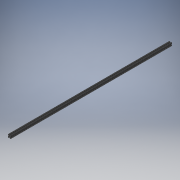
# Autodesk Inventor part: 30-3030-1708-CL
Saved by Autodesk Inventor 2019 (Build 230136000, 136)
## iProperties
Created: 2023-03-27
Part Number: 30-3030-1708-CL
Material: Generic
Catalog Web Link: www.cadenas.de
Description: 30-3030, 30-3030-Black-T-Slotted Profile - 30 Series
Vendor: 8020
Document SubType Name: Modeling
Designer: psAdmin
Manufacturer: 8020
Mass: 538.109 g
Surface Area: 5681.46 cm^2
Volume: 538.109 cm^3
Density: 1 g/cm^3
Appearance: PSOLRGB-191-191-191
Category: PARTsolutions
Company: 8020
Title: 30-3030-1708
Author: Cadenas PARTsolutions
Comments: T-Slotted Profile - 30 Series
PSOL_IDENT_0: {$CADENAS_DATA/23d-libs/8020/metric/profiles/30_series/30_3030.prj},192 {VTYP=3D},{NB=30-3030-1708-C
PSOL_IDENT_1: L},{LINA=30-3030-1708},{NN=30-3030, 30-3030-Black},{DATE=31.07.2020 09:21:33},{GEOMDATE=01.11.2018 1
PSOL_IDENT_2: 7:26:00},{VERSION=},{LINEID=10},{WBVAR=FIN,LS,L},{WBNUMERIC=L}  {NB=30-3030-1708-CL},{LINA=30-3030-1
PSOL_IDENT_3: 708},{KT=DUMMY},{PN=30-3030-1708},{PN1=30-3030},{FIN=CA},{LS=-CL},{L=1708.00},{SERIES=30-3030},{MAT=
PSOL_IDENT_4: 6105-T5 Aluminum},{W=0.9376},{LALG=[25:6000/0.05]},{MIX=2.7222},{MIY=2.7222},{EA=3.0877},{COLOR=.75,
PSOL_IDENT_5: .75,.75}
NB: 30-3030-1708-CL
NN: 30-3030, 30-3030-Black
NT: T-Slotted Profile - 30 Series
NBSYN: $PN.$LS.
LINA: 30-3030-1708
CATALOG: 80/20
PN: 30-3030-1708
FIN: Clear Anodize
LS: Custom Length
L: 1708
SERIES: 30-3030
MAT: 6105-T5 Aluminum
W: 0.9376
MIX: 2.7222
MIY: 2.7222
EA: 3.0877
SUPPLIER: 8020
ARTICLENO: 30-3030-1708-CL
BOMINFO: 30-3030-1708
CREATOR: CADENAS GmbH
Autodesk Inventor part; units mm, degrees
ref_plane "YZ Plane" through (0, 0, 0) normal (1, 0, 0) x (0, 1, 0)
ref_plane "XZ Plane" through (0, 0, 0) normal (0, 1, 0) x (-1, 0, 0)
ref_plane "XY Plane" through (0, 0, 0) normal (0, 0, 1) x (1, 0, 0)
sketch "Sketch_1" plane through (0, 0, 0) normal (0, 0, 1) x (1, 0, 0)
  arc A0 (-15, -13) -> (-13, -15) centre (-13, -13) ccw
  line L0 (-13, -15) -> (-4.508, -15)
  arc A1 (-4.508, -15) -> (-4, -14.492) centre (-4.508, -14.492) ccw
  line L1 (-4, -14.492) -> (-4, -13.251)
  arc A2 (-4, -13.251) -> (-4.508, -12.743) centre (-4.508, -13.251) ccw
  line L2 (-4.508, -12.743) -> (-7.742, -12.743)
  arc A3 (-8.25, -12.235) -> (-7.742, -12.743) centre (-7.742, -12.235) ccw
  line L3 (-8.25, -12.235) -> (-8.25, -10.2642)
  arc A4 (-8.1012, -9.905) -> (-8.25, -10.2642) centre (-7.742, -10.2642) ccw
  line L4 (-8.1012, -9.905) -> (-4.1795, -5.9833)
  arc A5 (-3.8203, -5.8345) -> (-4.1795, -5.9833) centre (-3.8203, -6.3425) ccw
  line L5 (-3.8203, -5.8345) -> (-0.949, -5.8345)
  line L6 (-0.949, -5.8345) -> (0, -5.325)
  line L7 (0, -5.325) -> (0.949, -5.8345)
  line L8 (0.949, -5.8345) -> (3.8216, -5.8345)
  arc A6 (4.1808, -5.9833) -> (3.8216, -5.8345) centre (3.8216, -6.3425) ccw
  line L9 (4.1808, -5.9833) -> (8.1012, -9.9037)
  arc A7 (8.25, -10.2629) -> (8.1012, -9.9037) centre (7.742, -10.2629) ccw
  line L10 (8.25, -10.2629) -> (8.25, -12.235)
  arc A8 (7.742, -12.743) -> (8.25, -12.235) centre (7.742, -12.235) ccw
  line L11 (7.742, -12.743) -> (4.508, -12.743)
  arc A9 (4.508, -12.743) -> (4, -13.251) centre (4.508, -13.251) ccw
  line L12 (4, -13.251) -> (4, -14.492)
  arc A10 (4, -14.492) -> (4.508, -15) centre (4.508, -14.492) ccw
  line L13 (4.508, -15) -> (13, -15)
  arc A11 (13, -15) -> (15, -13) centre (13, -13) ccw
  line L14 (15, -13) -> (15, -4.508)
  arc A12 (15, -4.508) -> (14.492, -4) centre (14.492, -4.508) ccw
  line L15 (14.492, -4) -> (13.251, -4)
  arc A13 (13.251, -4) -> (12.743, -4.508) centre (13.251, -4.508) ccw
  line L16 (12.743, -4.508) -> (12.743, -7.742)
  arc A14 (12.235, -8.25) -> (12.743, -7.742) centre (12.235, -7.742) ccw
  line L17 (12.235, -8.25) -> (10.2642, -8.25)
  arc A15 (9.905, -8.1012) -> (10.2642, -8.25) centre (10.2642, -7.742) ccw
  line L18 (9.905, -8.1012) -> (5.9833, -4.1795)
  arc A16 (5.8345, -3.8203) -> (5.9833, -4.1795) centre (6.3425, -3.8203) ccw
  line L19 (5.8345, -3.8203) -> (5.8345, -0.949)
  line L20 (5.8345, -0.949) -> (5.325, 0)
  line L21 (5.325, 0) -> (5.8345, 0.949)
  line L22 (5.8345, 0.949) -> (5.8345, 3.8216)
  arc A17 (5.9833, 4.1808) -> (5.8345, 3.8216) centre (6.3425, 3.8216) ccw
  line L23 (5.9833, 4.1808) -> (9.9037, 8.1012)
  arc A18 (10.2629, 8.25) -> (9.9037, 8.1012) centre (10.2629, 7.742) ccw
  line L24 (10.2629, 8.25) -> (12.235, 8.25)
  arc A19 (12.743, 7.742) -> (12.235, 8.25) centre (12.235, 7.742) ccw
  line L25 (12.743, 7.742) -> (12.743, 4.508)
  arc A20 (12.743, 4.508) -> (13.251, 4) centre (13.251, 4.508) ccw
  line L26 (13.251, 4) -> (14.492, 4)
  arc A21 (14.492, 4) -> (15, 4.508) centre (14.492, 4.508) ccw
  line L27 (15, 4.508) -> (15, 13)
  arc A22 (15, 13) -> (13, 15) centre (13, 13) ccw
  line L28 (13, 15) -> (4.508, 15)
  arc A23 (4.508, 15) -> (4, 14.492) centre (4.508, 14.492) ccw
  line L29 (4, 14.492) -> (4, 13.251)
  arc A24 (4, 13.251) -> (4.508, 12.743) centre (4.508, 13.251) ccw
  line L30 (4.508, 12.743) -> (7.742, 12.743)
  arc A25 (8.25, 12.235) -> (7.742, 12.743) centre (7.742, 12.235) ccw
  line L31 (8.25, 12.235) -> (8.25, 10.2642)
  arc A26 (8.1012, 9.905) -> (8.25, 10.2642) centre (7.742, 10.2642) ccw
  line L32 (8.1012, 9.905) -> (4.1795, 5.9833)
  arc A27 (3.8203, 5.8345) -> (4.1795, 5.9833) centre (3.8203, 6.3425) ccw
  line L33 (3.8203, 5.8345) -> (0.949, 5.8345)
  line L34 (0.949, 5.8345) -> (0, 5.325)
  line L35 (0, 5.325) -> (-0.949, 5.8345)
  line L36 (-0.949, 5.8345) -> (-3.8216, 5.8345)
  arc A28 (-4.1808, 5.9833) -> (-3.8216, 5.8345) centre (-3.8216, 6.3425) ccw
  line L37 (-4.1808, 5.9833) -> (-8.1012, 9.9037)
  arc A29 (-8.25, 10.2629) -> (-8.1012, 9.9037) centre (-7.742, 10.2629) ccw
  line L38 (-8.25, 10.2629) -> (-8.25, 12.235)
  arc A30 (-7.742, 12.743) -> (-8.25, 12.235) centre (-7.742, 12.235) ccw
  line L39 (-7.742, 12.743) -> (-4.508, 12.743)
  arc A31 (-4.508, 12.743) -> (-4, 13.251) centre (-4.508, 13.251) ccw
  line L40 (-4, 13.251) -> (-4, 14.492)
  arc A32 (-4, 14.492) -> (-4.508, 15) centre (-4.508, 14.492) ccw
  line L41 (-4.508, 15) -> (-13, 15)
  arc A33 (-13, 15) -> (-15, 13) centre (-13, 13) ccw
  line L42 (-15, 13) -> (-15, 4.508)
  arc A34 (-15, 4.508) -> (-14.492, 4) centre (-14.492, 4.508) ccw
  line L43 (-14.492, 4) -> (-13.251, 4)
  arc A35 (-13.251, 4) -> (-12.743, 4.508) centre (-13.251, 4.508) ccw
  line L44 (-12.743, 4.508) -> (-12.743, 7.742)
  arc A36 (-12.235, 8.25) -> (-12.743, 7.742) centre (-12.235, 7.742) ccw
  line L45 (-12.235, 8.25) -> (-10.2642, 8.25)
  arc A37 (-9.905, 8.1012) -> (-10.2642, 8.25) centre (-10.2642, 7.742) ccw
  line L46 (-9.905, 8.1012) -> (-5.9833, 4.1795)
  arc A38 (-5.8345, 3.8203) -> (-5.9833, 4.1795) centre (-6.3425, 3.8203) ccw
  line L47 (-5.8345, 3.8203) -> (-5.8345, 0.949)
  line L48 (-5.8345, 0.949) -> (-5.325, 0)
  line L49 (-5.325, 0) -> (-5.8345, -0.949)
  line L50 (-5.8345, -0.949) -> (-5.8345, -3.8216)
  arc A39 (-5.9833, -4.1808) -> (-5.8345, -3.8216) centre (-6.3425, -3.8216) ccw
  line L51 (-5.9833, -4.1808) -> (-9.9037, -8.1012)
  arc A40 (-10.2629, -8.25) -> (-9.9037, -8.1012) centre (-10.2629, -7.742) ccw
  line L52 (-10.2629, -8.25) -> (-12.235, -8.25)
  arc A41 (-12.743, -7.742) -> (-12.235, -8.25) centre (-12.235, -7.742) ccw
  line L53 (-12.743, -7.742) -> (-12.743, -4.508)
  arc A42 (-12.743, -4.508) -> (-13.251, -4) centre (-13.251, -4.508) ccw
  line L54 (-13.251, -4) -> (-14.492, -4)
  arc A43 (-14.492, -4) -> (-15, -4.508) centre (-14.492, -4.508) ccw
  line L55 (-15, -4.508) -> (-15, -13)
  arc A44 (9.5, -13.319) -> (9.881, -13.7) centre (9.881, -13.319) ccw
  line L56 (9.881, -13.7) -> (12.7, -13.7)
  arc A45 (12.7, -13.7) -> (13.7, -12.7) centre (12.7, -12.7) ccw
  line L57 (13.7, -12.7) -> (13.7, -9.881)
  arc A46 (13.7, -9.881) -> (13.319, -9.5) centre (13.319, -9.881) ccw
  line L58 (13.319, -9.5) -> (9.881, -9.5)
  arc A47 (9.881, -9.5) -> (9.5, -9.881) centre (9.881, -9.881) ccw
  line L59 (9.5, -9.881) -> (9.5, -13.319)
  arc A48 (9.5, 9.881) -> (9.881, 9.5) centre (9.881, 9.881) ccw
  line L60 (9.881, 9.5) -> (13.319, 9.5)
  arc A49 (13.319, 9.5) -> (13.7, 9.881) centre (13.319, 9.881) ccw
  line L61 (13.7, 9.881) -> (13.7, 12.7)
  arc A50 (13.7, 12.7) -> (12.7, 13.7) centre (12.7, 12.7) ccw
  line L62 (12.7, 13.7) -> (9.881, 13.7)
  arc A51 (9.881, 13.7) -> (9.5, 13.319) centre (9.881, 13.319) ccw
  line L63 (9.5, 13.319) -> (9.5, 9.881)
  arc A52 (-4.0107, -2.5139) -> (-2.5139, -4.0107) centre (-3.142, -3.142) ccw
  line L64 (-2.5139, -4.0107) -> (-1.3138, -3.0544)
  arc A53 (-1.3138, -3.0544) -> (1.3138, -3.0544) centre (0, 0) ccw
  line L65 (1.3138, -3.0544) -> (2.5139, -4.0107)
  arc A54 (2.5139, -4.0107) -> (4.0107, -2.5139) centre (3.142, -3.142) ccw
  line L66 (4.0107, -2.5139) -> (3.0544, -1.3138)
  arc A55 (3.0544, -1.3138) -> (3.0544, 1.3138) centre (0, 0) ccw
  line L67 (3.0544, 1.3138) -> (4.0107, 2.5139)
  arc A56 (4.0107, 2.5139) -> (2.5139, 4.0107) centre (3.142, 3.142) ccw
  line L68 (2.5139, 4.0107) -> (1.3138, 3.0544)
  arc A57 (1.3138, 3.0544) -> (-1.3138, 3.0544) centre (0, 0) ccw
  line L69 (-1.3138, 3.0544) -> (-2.5139, 4.0107)
  arc A58 (-2.5139, 4.0107) -> (-4.0107, 2.5139) centre (-3.142, 3.142) ccw
  line L70 (-4.0107, 2.5139) -> (-3.0544, 1.3138)
  arc A59 (-3.0544, 1.3138) -> (-3.0544, -1.3138) centre (0, 0) ccw
  line L71 (-3.0544, -1.3138) -> (-4.0107, -2.5139)
  arc A60 (-13.7, 9.881) -> (-13.319, 9.5) centre (-13.319, 9.881) ccw
  line L72 (-13.319, 9.5) -> (-9.881, 9.5)
  arc A61 (-9.881, 9.5) -> (-9.5, 9.881) centre (-9.881, 9.881) ccw
  line L73 (-9.5, 9.881) -> (-9.5, 13.319)
  arc A62 (-9.5, 13.319) -> (-9.881, 13.7) centre (-9.881, 13.319) ccw
  line L74 (-9.881, 13.7) -> (-12.7, 13.7)
  arc A63 (-12.7, 13.7) -> (-13.7, 12.7) centre (-12.7, 12.7) ccw
  line L75 (-13.7, 12.7) -> (-13.7, 9.881)
  arc A64 (-13.7, -12.7) -> (-12.7, -13.7) centre (-12.7, -12.7) ccw
  line L76 (-12.7, -13.7) -> (-9.881, -13.7)
  arc A65 (-9.881, -13.7) -> (-9.5, -13.319) centre (-9.881, -13.319) ccw
  line L77 (-9.5, -13.319) -> (-9.5, -9.881)
  arc A66 (-9.5, -9.881) -> (-9.881, -9.5) centre (-9.881, -9.881) ccw
  line L78 (-9.881, -9.5) -> (-13.319, -9.5)
  arc A67 (-13.319, -9.5) -> (-13.7, -9.881) centre (-13.319, -9.881) ccw
  line L79 (-13.7, -9.881) -> (-13.7, -12.7)
  constraints: 160 end point, 136 point on circle, 68 centre point
extrude "Extrusion1" add sketch "Sketch_1" against normal blind 1708
body "Solid1"
